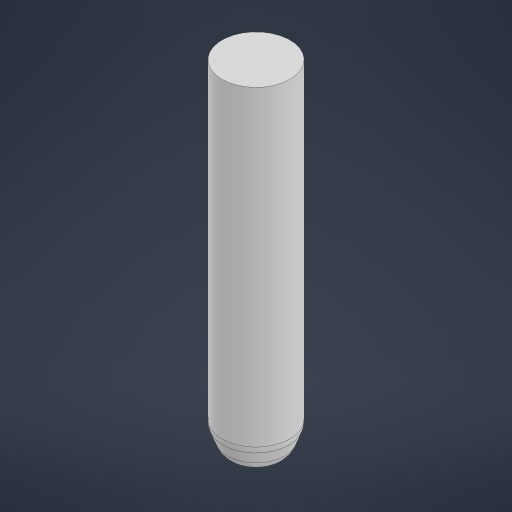
# Autodesk Inventor part: M4_dowel_pin
Saved by Autodesk Inventor 2024.2 (Build 282272000, 272)
## iProperties
Created: 2026-01-04
Part Number: M4_dowel_pin
Material: Generic
Document SubType Name: Modeling
Designer: 4aida
Density: 1 g/cm^3
Appearance: Default
Author: 4aida
Autodesk Inventor part; units mm, degrees
ref_plane "YZ Plane" through (0, 0, 0) normal (1, 0, 0) x (0, 1, 0)
ref_plane "XZ Plane" through (0, 0, 0) normal (0, 1, 0) x (-1, 0, 0)
ref_plane "XY Plane" through (0, 0, 0) normal (0, 0, 1) x (1, 0, 0)
sketch "Sketch1" plane through (0, 0, 0) normal (0, 0, 1) x (1, 0, 0)
  line L0 (2, 10) -> (2, -8.5)
  line L1 (2, -8.5) -> (1.454, -10)
  line L2 (1.454, -10) -> (0, -10)
  line L3 (0, -10) -> (0, 10)
  line L4 (0, 10) -> (2, 10)
  point P0 (0, 0)
  point P1 (0, 0)
  dimension "d0" = 4
  dimension "d1" = 20
  dimension "d2" = 160
  dimension "d3" = 1.5
  constraints: 10 end point, 3 perpendicular, 1 coincident, 1 midpoint, 1 vertical
  measures "d0" diameter of L0 L3
  measures "d1" distance of L2.end L3.end
  measures "d2" angle of L0 L1
  measures "d3" vertical distance of L0.end L1.end
revolve "Revolution1" add sketch "Sketch1" angle 360 about axis through (0, -10, 0) along (0, 1, 0)
fillet "Fillet1" radius 1 2 edges at (-1.454, -10, 0) (-2, -8.5, 0)
body "Solid1"
